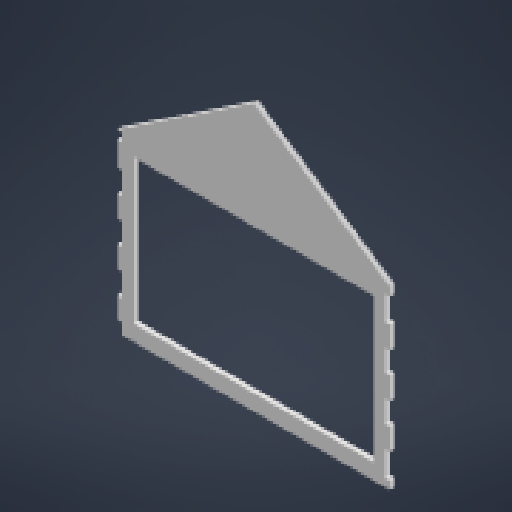
# Autodesk Inventor part: Pieza4
Saved by Autodesk Inventor 2026.1 (Build 301233020, 233B)
## iProperties
Created: 2026-05-06
Part Number: Pieza4
Material: Genérico
Document SubType Name: Modeling
Designer: OlmesTech
Density: 1 g/cm^3
Appearance: Valor por defecto
Author: OlmesTech
Autodesk Inventor part; units mm, degrees
ref_plane "YZ Plane" through (0, 0, 0) normal (1, 0, 0) x (0, 1, 0)
ref_plane "XZ Plane" through (0, 0, 0) normal (0, 1, 0) x (-1, 0, 0)
ref_plane "XY Plane" through (0, 0, 0) normal (0, 0, 1) x (1, 0, 0)
sketch "Boceto1" plane through (0, 0, 0) normal (0, 0, 1) x (1, 0, 0)
  line L0 (0, 3) -> (170, 3) projected
  line L1 (0, 113) -> (170, 113)
  line L2 (10, 103) -> (10, 13)
  line L3 (10, 13) -> (160, 13)
  line L4 (160, 13) -> (160, 103)
  line L5 (10, 103) -> (160, 103)
  line L6 (85, 169.6763) -> (0, 113)
  line L7 (85, 169.6763) -> (170, 113)
  line L8 (0, 92.5) -> (0, 107.7321) projected
  line L9 (0, 92.5) -> (3, 92.5) projected
  line L10 (3, 107.7321) -> (3, 92.5) projected
  line L11 (0, 107.7321) -> (3, 107.7321) projected
  line L12 (3, 113) -> (3, 107.7321) projected
  line L13 (3, 92.5) -> (3, 78.5) projected
  line L14 (0, 65) -> (0, 78.5) projected
  line L15 (0, 65) -> (3, 65) projected
  line L16 (3, 78.5) -> (3, 65) projected
  line L17 (0, 78.5) -> (3, 78.5) projected
  line L18 (3, 65) -> (3, 51) projected
  line L19 (0, 37.5) -> (0, 51) projected
  line L20 (0, 37.5) -> (3, 37.5) projected
  line L21 (3, 51) -> (3, 37.5) projected
  line L22 (0, 51) -> (3, 51) projected
  line L23 (3, 37.5) -> (3, 23.5) projected
  line L24 (0, 10) -> (0, 23.5) projected
  line L25 (0, 10) -> (3, 10) projected
  line L26 (3, 23.5) -> (3, 10) projected
  line L27 (0, 23.5) -> (3, 23.5) projected
  line L28 (3, 10) -> (3, 3) projected
  line L29 (170, 113) -> (170, 107.7321) projected
  line L30 (170, 113) -> (167, 113) projected
  line L31 (167, 107.7321) -> (167, 113) projected
  line L32 (170, 107.7321) -> (167, 107.7321) projected
  line L33 (167, 92.5) -> (167, 107.7321) projected
  line L34 (170, 92.5) -> (170, 78.5) projected
  line L35 (170, 92.5) -> (167, 92.5) projected
  line L36 (167, 78.5) -> (167, 92.5) projected
  line L37 (170, 78.5) -> (167, 78.5) projected
  line L38 (167, 65) -> (167, 78.5) projected
  line L39 (170, 65) -> (170, 51) projected
  line L40 (170, 65) -> (167, 65) projected
  line L41 (167, 51) -> (167, 65) projected
  line L42 (170, 51) -> (167, 51) projected
  line L43 (167, 37.5) -> (167, 51) projected
  line L44 (170, 37.5) -> (170, 23.5) projected
  line L45 (170, 37.5) -> (167, 37.5) projected
  line L46 (167, 23.5) -> (167, 37.5) projected
  line L47 (170, 23.5) -> (167, 23.5) projected
  line L48 (167, 8.2679) -> (167, 23.5) projected
  line L49 (170, 8.2679) -> (170, 3) projected
  line L50 (170, 8.2679) -> (167, 8.2679) projected
  line L51 (167, 3) -> (167, 8.2679) projected
  line L52 (170, 3) -> (167, 3) projected
  point P0 (0, 0)
  point P1 (86.5, 171.1763)
  point P2 (83.5, 171.1763)
  dimension "d0" = 110
  dimension "d8" = 10
  constraints: 14 end point, 1 horizontal, 1 parallel
  measures "d0" distance of L0.start L1.start
  measures "d8" distance between parallel lines of L1 L5
extrude "Extrusión1" add sketch "Boceto1" against normal blind 3
